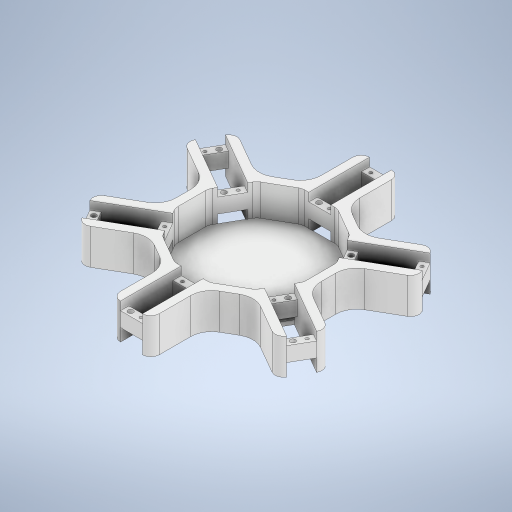
# Autodesk Inventor part: HexBodyBottom
Saved by Autodesk Inventor 2024 (Build 280153000, 153)
## iProperties
Created: 2026-02-25
Part Number: HexBodyBottom
Material: Generic
Document SubType Name: Modeling
Designer: Liam
Density: 1 g/cm^3
Appearance: Default
Author: Liam
Autodesk Inventor part; units mm, degrees
ref_plane "YZ Plane" through (0, 0, 0) normal (1, 0, 0) x (0, 1, 0)
ref_plane "XZ Plane" through (0, 0, 0) normal (0, 1, 0) x (-1, 0, 0)
ref_plane "XY Plane" through (0, 0, 0) normal (0, 0, 1) x (1, 0, 0)
sketch "Sketch1" plane through (0, 0, 0) normal (0, 1, 0) x (-1, 0, 0)
  line L0 (0, -80) -> (-69.282, -40)
  line L1 (-69.282, -40) -> (-69.282, 40)
  line L2 (-69.282, 40) -> (0, 80)
  line L3 (0, 80) -> (69.282, 40)
  line L4 (69.282, 40) -> (69.282, -40)
  line L5 (69.282, -40) -> (0, -80)
  line L6 (128, 128) -> (-128, 128)
  line L7 (-128, 128) -> (-128, -128)
  line L8 (-128, -128) -> (128, -128)
  line L9 (128, -128) -> (128, 128)
  line L10 (128, 128) -> (-128, -128) construction
  line L11 (-128, 128) -> (128, -128) construction
  line L12 (10.5, 111) -> (-10.5, 111)
  line L13 (-10.5, 111) -> (-10.5, 69)
  line L14 (-10.5, 69) -> (10.5, 69)
  line L15 (10.5, 69) -> (10.5, 111)
  line L16 (10.5, 111) -> (-10.5, 69) construction
  line L17 (-10.5, 111) -> (10.5, 69) construction
  line L18 (18.5, 119) -> (-18.5, 119)
  line L19 (-18.5, 119) -> (-18.5, 61)
  line L20 (-18.5, 61) -> (18.5, 61)
  line L21 (18.5, 61) -> (18.5, 119)
  line L22 (61.282, 35.3812) -> (0, 70.7624)
  line L23 (0, 70.7624) -> (-61.282, 35.3812)
  line L24 (-61.282, 35.3812) -> (-61.282, -35.3812)
  line L25 (-61.282, -35.3812) -> (0, -70.7624)
  line L26 (0, -70.7624) -> (61.282, -35.3812)
  line L27 (61.282, -35.3812) -> (61.282, 35.3812)
  circle A0 centre (-5, 114.75) radius 1.5
  circle A1 centre (5, 114.75) radius 2.5
  circle A2 centre (5, 65.25) radius 1.5
  circle A3 centre (-5, 65.25) radius 2.5
  line L28 (-10.5, 111) -> (-10.5, 119)
  line L29 (10.5, 111) -> (10.5, 119)
  line L30 (-10.5, 69) -> (-10.5, 61)
  line L31 (10.5, 69) -> (10.5, 61)
  line L32 (-43.5775, 46.5215) -> (-93.807, 75.5215)
  line L33 (-93.807, 75.5215) -> (-112.307, 43.4785)
  line L34 (-90.8788, 64.5933) -> (-97.807, 68.5933)
  line L35 (-54.5058, 43.5933) -> (-90.8788, 64.5933)
  line L36 (-90.8788, 64.5933) -> (-101.3788, 46.4067)
  circle A4 centre (-96.8764, 61.7051) radius 2.5
  circle A5 centre (-101.8764, 53.0449) radius 1.5
  line L37 (-101.3788, 46.4067) -> (-108.307, 50.4067)
  line L38 (-101.3788, 46.4067) -> (-65.0058, 25.4067)
  line L39 (-112.307, 43.4785) -> (-62.0775, 14.4785)
  line L40 (-62.0775, 14.4785) -> (-43.5775, 46.5215)
  line L41 (-65.0058, 25.4067) -> (-58.0775, 21.4067)
  circle A6 centre (-59.0082, 28.2949) radius 2.5
  circle A7 centre (-54.0082, 36.9551) radius 1.5
  line L42 (-65.0058, 25.4067) -> (-54.5058, 43.5933)
  line L43 (-54.5058, 43.5933) -> (-47.5775, 39.5933)
  line L44 (-62.0775, -14.4785) -> (-112.307, -43.4785)
  line L45 (-112.307, -43.4785) -> (-93.807, -75.5215)
  line L46 (-101.3788, -46.4067) -> (-108.307, -50.4067)
  line L47 (-65.0058, -25.4067) -> (-101.3788, -46.4067)
  line L48 (-101.3788, -46.4067) -> (-90.8788, -64.5933)
  circle A8 centre (-101.8764, -53.0449) radius 2.5
  circle A9 centre (-96.8764, -61.7051) radius 1.5
  line L49 (-90.8788, -64.5933) -> (-97.807, -68.5933)
  line L50 (-90.8788, -64.5933) -> (-54.5058, -43.5933)
  line L51 (-93.807, -75.5215) -> (-43.5775, -46.5215)
  line L52 (-43.5775, -46.5215) -> (-62.0775, -14.4785)
  line L53 (-54.5058, -43.5933) -> (-47.5775, -39.5933)
  circle A10 centre (-54.0082, -36.9551) radius 2.5
  circle A11 centre (-59.0082, -28.2949) radius 1.5
  line L54 (-54.5058, -43.5933) -> (-65.0058, -25.4067)
  line L55 (-65.0058, -25.4067) -> (-58.0775, -21.4067)
  line L56 (-18.5, -61) -> (-18.5, -119)
  line L57 (-18.5, -119) -> (18.5, -119)
  line L58 (-10.5, -111) -> (-10.5, -119)
  line L59 (-10.5, -69) -> (-10.5, -111)
  line L60 (-10.5, -111) -> (10.5, -111)
  circle A12 centre (-5, -114.75) radius 2.5
  circle A13 centre (5, -114.75) radius 1.5
  line L61 (10.5, -111) -> (10.5, -119)
  line L62 (10.5, -111) -> (10.5, -69)
  line L63 (18.5, -119) -> (18.5, -61)
  line L64 (18.5, -61) -> (-18.5, -61)
  line L65 (10.5, -69) -> (10.5, -61)
  circle A14 centre (5, -65.25) radius 2.5
  circle A15 centre (-5, -65.25) radius 1.5
  line L66 (10.5, -69) -> (-10.5, -69)
  line L67 (-10.5, -69) -> (-10.5, -61)
  line L68 (43.5775, -46.5215) -> (93.807, -75.5215)
  line L69 (93.807, -75.5215) -> (112.307, -43.4785)
  line L70 (90.8788, -64.5933) -> (97.807, -68.5933)
  line L71 (54.5058, -43.5933) -> (90.8788, -64.5933)
  line L72 (90.8788, -64.5933) -> (101.3788, -46.4067)
  circle A16 centre (96.8764, -61.7051) radius 2.5
  circle A17 centre (101.8764, -53.0449) radius 1.5
  line L73 (101.3788, -46.4067) -> (108.307, -50.4067)
  line L74 (101.3788, -46.4067) -> (65.0058, -25.4067)
  line L75 (112.307, -43.4785) -> (62.0775, -14.4785)
  line L76 (62.0775, -14.4785) -> (43.5775, -46.5215)
  line L77 (65.0058, -25.4067) -> (58.0775, -21.4067)
  circle A18 centre (59.0082, -28.2949) radius 2.5
  circle A19 centre (54.0082, -36.9551) radius 1.5
  line L78 (65.0058, -25.4067) -> (54.5058, -43.5933)
  line L79 (54.5058, -43.5933) -> (47.5775, -39.5933)
  line L80 (62.0775, 14.4785) -> (112.307, 43.4785)
  line L81 (112.307, 43.4785) -> (93.807, 75.5215)
  line L82 (101.3788, 46.4067) -> (108.307, 50.4067)
  line L83 (65.0058, 25.4067) -> (101.3788, 46.4067)
  line L84 (101.3788, 46.4067) -> (90.8788, 64.5933)
  circle A20 centre (101.8764, 53.0449) radius 2.5
  circle A21 centre (96.8764, 61.7051) radius 1.5
  line L85 (90.8788, 64.5933) -> (97.807, 68.5933)
  line L86 (90.8788, 64.5933) -> (54.5058, 43.5933)
  line L87 (93.807, 75.5215) -> (43.5775, 46.5215)
  line L88 (43.5775, 46.5215) -> (62.0775, 14.4785)
  line L89 (54.5058, 43.5933) -> (47.5775, 39.5933)
  circle A22 centre (54.0082, 36.9551) radius 2.5
  circle A23 centre (59.0082, 28.2949) radius 1.5
  line L90 (54.5058, 43.5933) -> (65.0058, 25.4067)
  line L91 (65.0058, 25.4067) -> (58.0775, 21.4067)
  point P0 (0, 0)
  point P1 (0, 0)
  point P2 (0, 0)
  point P3 (0, 90)
  point P4 (30.641, 53.0718)
  point P5 (0, 69)
  point P6 (16.909, 61)
  point P7 (-16.909, 61)
  point P8 (-18.5, 69.319)
  point P9 (18.5, 69.319)
  point P10 (-59.7558, 34.5)
  point P11 (-59.7558, -34.5)
  point P12 (0, -69)
  point P13 (59.7558, -34.5)
  point P14 (59.7558, 34.5)
  point P15 (-69.282, 18.638)
  point P16 (-69.282, -18.638)
  point P17 (-50.782, -50.681)
  point P18 (-18.5, -69.319)
  point P19 (18.5, -69.319)
  point P20 (50.782, -50.681)
  point P21 (69.282, -18.638)
  point P22 (69.282, 18.638)
  point P23 (50.782, 50.681)
  point P24 (44.3731, 45.1436)
  point P25 (61.282, 15.8564)
  point P26 (61.282, -15.8564)
  point P27 (44.3731, -45.1436)
  point P28 (16.909, -61)
  point P29 (-16.909, -61)
  point P30 (-44.3731, -45.1436)
  point P31 (-61.282, -15.8564)
  point P32 (-61.282, 15.8564)
  point P33 (-44.3731, 45.1436)
  point P34 (-50.782, 50.681)
  point P35 (10.5, 73.9378)
  point P36 (-10.5, 73.9378)
  point P37 (-58.782, 46.0622)
  point P38 (-69.282, 27.8756)
  point P39 (-69.282, -27.8756)
  point P40 (-58.782, -46.0622)
  point P41 (-10.5, -73.9378)
  point P42 (10.5, -73.9378)
  point P43 (58.782, -46.0622)
  point P44 (69.282, -27.8756)
  point P45 (69.282, 27.8756)
  point P46 (58.782, 46.0622)
  dimension "d0" = 0
  dimension "d1" = 80
  dimension "d2" = 256
  dimension "d3" = 256
  dimension "d4" = 0
  dimension "d5" = 0
  dimension "d7" = 90
  dimension "d9" = 0
  dimension "d10" = 42
  dimension "d11" = 21
  dimension "d12" = 8
  dimension "d13" = 8
  dimension "d14" = 119
  dimension "d15" = 3
  dimension "d16" = 5
  dimension "d17" = 3.75
  dimension "d18" = 3.75
  dimension "d19" = 5
  dimension "d20" = 5
  dimension "d21" = 3
  dimension "d22" = 5
  dimension "d23" = 3.75
  dimension "d24" = 3.75
  dimension "d25" = 5
  dimension "d26" = 5
  dimension "d37" = 360
  constraints: 184 end point, 30 point on line, 24 centre point, 6 midpoint, 6 parallel, 6 perpendicular, 2 horizontal, 1 coincident, 220 other
  measures "d0" horizontal distance of L0.start point (0, 0)
  measures "d1" distance of L3.end L4.end
  measures "d2" distance of L6.start L6.end
  measures "d3" distance of L6.end L7.end
  measures "d4" distance of point (0, 0) point (0, 0)
  measures "d5" distance of point (0, 0) point (0, 0)
  measures "d7" distance of point (0, 0) point (0, 90)
  measures "d9" horizontal distance of L2.end point (0, 90)
  measures "d10" distance of L14.end L12.start
  measures "d11" distance of L13.end L14.end
  measures "d12" distance between parallel lines of L21 L15
  measures "d13" distance from line of point (30.641, 53.072) L3
  measures "d14" distance from line of point (0, 0) L18
  measures "d15" diameter of A0
  measures "d16" diameter of A1
  measures "d17" distance from line of L12 A1.centre
  measures "d18" distance from line of L12 A0.centre
  measures "d19" horizontal distance of point (0, 90) A0.centre
  measures "d20" horizontal distance of A1.centre point (0, 90)
  measures "d21" diameter of A2
  measures "d22" diameter of A3
  measures "d23" distance from line of L14 A3.centre
  measures "d24" distance from line of L14 A2.centre
  measures "d25" horizontal distance of point (0, 69) A2.centre
  measures "d26" horizontal distance of point (0, 69) A3.centre
extrude "Extrusion1" add sketch "Sketch1" along normal blind 22 contours L59 L58 L57 L56 L0 | L0 L56 L64 L25 L67 L59 | L62 L65 L26 L64 L63 L5 | L5 L63 L57 L61 L62 | L0 L51 L52 L25 L64 L56 | L67 L25 L66 | L60 L61 L57 L58 | L63 L64 L26 L76 L68 L5 | L66 L26 A14 L65 | L51 L45 L49 L50 L0 | L0 L50 L53 L25 L52 L51 | L25 L67 L64 L65 L26 A14 L66 | L25 L64 L67 | L68 L76 L26 L79 L71 L5 | L5 L71 L70 L69 L68 | L65 L64 L26 | L49 L45 L46 L48 | L54 L25 A10 L53 | L25 L53 L52 | L79 L26 L78 | L72 L73 L69 L70 | L76 L79 L26 | L47 L46 L45 L44 L1 | L1 L44 L52 L24 L55 L47 | L25 A10 L54 L24 L55 L52 L53 | L74 L77 L27 L76 L75 L4 | L4 L75 L69 L73 L74 | L26 L79 L76 L77 L27 A18 L78 | L1 L39 L40 L24 L52 L44 | L55 L24 L54 | L55 L24 L52 | L75 L76 L27 L88 L80 L4 | L78 L27 A18 L77 | L76 L27 L77 | L39 L33 L37 L38 L1 | L1 L38 L41 L24 L40 L39 | L80 L88 L27 L91 L83 L4 | L4 L83 L82 L81 L80 | L24 L41 L40 | L88 L91 L27 | L37 L33 L34 L36 | L42 L24 A6 L41 | L24 A6 L42 L23 L43 L40 L41 | L91 L27 L90 | L84 L85 L81 L82 | L91 L88 L89 L22 A22 L90 L27 | L35 L34 L33 L32 L2 | L2 L32 L40 L23 L43 L35 | L43 L23 L40 | L86 L89 L22 L88 L87 L3 | L3 L87 L81 L85 L86 | L88 L22 L89 | L2 L19 L20 L23 L40 L32 | L43 L23 L42 | L87 L88 L22 L20 L21 L3 | L90 L22 A22 L89 | L19 L18 L28 L13 L2 | L2 L13 L30 L23 L20 L19 | L23 L30 L20 | L21 L20 L22 L31 L15 L3 | L3 L15 L29 L18 L21 | L20 L31 L22 | L30 L23 A3 L14 L22 L31 L20 | L30 L14 L23 A3 | L22 L14 L31 | L28 L18 L29 L12
extrude "Extrusion2" cut sketch "Sketch1" along normal blind 8 contours L67 L25 L66 | L60 L61 L57 L58 | L66 L26 A14 L65 | L25 L67 L64 L65 L26 A14 L66 | L49 L45 L46 L48 | L54 L25 A10 L53 | L79 L26 L78 | L72 L73 L69 L70 | L25 A10 L54 L24 L55 L52 L53 | L26 L79 L76 L77 L27 A18 L78 | L55 L24 L54 | L78 L27 A18 L77 | L37 L33 L34 L36 | L42 L24 A6 L41 | L24 A6 L42 L23 L43 L40 L41 | L91 L27 L90 | L84 L85 L81 L82 | L91 L88 L89 L22 A22 L90 L27 | L43 L23 L42 | L90 L22 A22 L89 | L30 L23 A3 L14 L22 L31 L20 | L30 L14 L23 A3 | L22 L14 L31 | L28 L18 L29 L12
extrude "Extrusion3" add sketch "Sketch1" against normal blind 4 contours L59 L58 L57 L56 L0 | L0 L56 L64 L25 L67 L59 | L62 L65 L26 L64 L63 L5 | L5 L63 L57 L61 L62 | L0 L51 L52 L25 L64 L56 | L63 L64 L26 L76 L68 L5 | L51 L45 L49 L50 L0 | L0 L50 L53 L25 L52 L51 | L25 L64 L67 | L68 L76 L26 L79 L71 L5 | L5 L71 L70 L69 L68 | L65 L64 L26 | L25 L52 L24 L40 L23 L20 L22 L88 L27 L76 L26 L64 | L25 L53 L52 | L76 L79 L26 | L47 L46 L45 L44 L1 | L1 L44 L52 L24 L55 L47 | L74 L77 L27 L76 L75 L4 | L4 L75 L69 L73 L74 | L1 L39 L40 L24 L52 L44 | L55 L24 L52 | L75 L76 L27 L88 L80 L4 | L76 L27 L77 | L39 L33 L37 L38 L1 | L1 L38 L41 L24 L40 L39 | L80 L88 L27 L91 L83 L4 | L4 L83 L82 L81 L80 | L24 L41 L40 | L88 L91 L27 | L35 L34 L33 L32 L2 | L2 L32 L40 L23 L43 L35 | L43 L23 L40 | L86 L89 L22 L88 L87 L3 | L3 L87 L81 L85 L86 | L88 L22 L89 | L2 L19 L20 L23 L40 L32 | L87 L88 L22 L20 L21 L3 | L19 L18 L28 L13 L2 | L2 L13 L30 L23 L20 L19 | L23 L30 L20 | L21 L20 L22 L31 L15 L3 | L3 L15 L29 L18 L21 | L20 L31 L22
extrude "Extrusion4" add sketch "Sketch1" along normal blind 30 contours L59 L58 L57 L56 L0 | L0 L56 L64 L25 L67 L59 | L62 L65 L26 L64 L63 L5 | L5 L63 L57 L61 L62 | L0 L51 L52 L25 L64 L56 | L63 L64 L26 L76 L68 L5 | L51 L45 L49 L50 L0 | L0 L50 L53 L25 L52 L51 | L25 L64 L67 | L68 L76 L26 L79 L71 L5 | L5 L71 L70 L69 L68 | L65 L64 L26 | L25 L53 L52 | L76 L79 L26 | L47 L46 L45 L44 L1 | L1 L44 L52 L24 L55 L47 | L74 L77 L27 L76 L75 L4 | L4 L75 L69 L73 L74 | L1 L39 L40 L24 L52 L44 | L55 L24 L52 | L75 L76 L27 L88 L80 L4 | L76 L27 L77 | L39 L33 L37 L38 L1 | L1 L38 L41 L24 L40 L39 | L80 L88 L27 L91 L83 L4 | L4 L83 L82 L81 L80 | L24 L41 L40 | L88 L91 L27 | L35 L34 L33 L32 L2 | L2 L32 L40 L23 L43 L35 | L43 L23 L40 | L86 L89 L22 L88 L87 L3 | L3 L87 L81 L85 L86 | L88 L22 L89 | L2 L19 L20 L23 L40 L32 | L87 L88 L22 L20 L21 L3 | L19 L18 L28 L13 L2 | L2 L13 L30 L23 L20 L19 | L23 L30 L20 | L21 L20 L22 L31 L15 L3 | L3 L15 L29 L18 L21 | L20 L31 L22
fillet "Fillet1" radius 8 12 edges at (-93.807, 13, 75.5215) (-112.307, 13, 43.4785) (18.5, 13, 119) (93.807, 13, 75.5215) (112.307, 13, 43.4785) (112.307, 13, -43.4785) (93.807, 13, -75.5215) (18.5, 13, -119) (-18.5, 13, -119) (-93.807, 13, -75.5215) (-112.307, 13, -43.4785) (-18.5, 13, 119)
fillet "Fillet2" radius 20 12 edges at (18.5, 13, 69.319) (50.782, 13, 50.681) (69.282, 13, 18.638) (69.282, 13, -18.638) (50.782, 13, -50.681) (18.5, 13, -69.319) (-18.5, 13, -69.319) (-50.782, 13, -50.681) (-69.282, 13, -18.638) (-69.282, 13, 18.638) (-50.782, 13, 50.681) (-18.5, 13, 69.319)
fillet "Fillet3" radius 10 12 edges at (61.282, 15, -15.8564) (61.282, 15, 15.8564) (44.3731, 15, 45.1436) (16.909, 15, 61) (-16.909, 15, 61) (-44.3731, 15, 45.1436) (-61.282, 15, 15.8564) (-61.282, 15, -15.8564) (-44.3731, 15, -45.1436) (-16.909, 15, -61) (16.909, 15, -61) (44.3731, 15, -45.1436)
equation "\"d10\" = MountLength"
equation "\"d11\" = MountWidth"
equation "\"d12\" = MountThickness"
equation "\"d13\" = MountThickness"
equation "\"d15\" = HOLE_DIAMETER"
equation "\"d16\" = INSERT_DIAMETER"
equation "\"d17\" = MountHoleY"
equation "\"d18\" = MountHoleY"
equation "\"d19\" = MountHoleX"
equation "\"d20\" = MountHoleX"
equation "\"d21\" = HOLE_DIAMETER"
equation "\"d22\" = INSERT_DIAMETER"
equation "\"d23\" = MountHoleY"
equation "\"d24\" = MountHoleY"
equation "\"d25\" = MountHoleX"
equation "\"d26\" = MountHoleX"
equation "\"d27\" = OUTER_HEIGHT + INNER_HEIGHT"
equation "\"d29\" = OUTER_HEIGHT"
equation "\"d33\" = 2 * OUTER_HEIGHT + INNER_HEIGHT"
equation "\"MountLength\" = 42"
equation "\"MountWidth\" = 21"
equation "\"MountThickness\" = 8"
equation "\"HOLE_DIAMETER\" = 3"
equation "\"INSERT_DIAMETER\" = 5"
equation "\"MountHoleY\" = 3.75"
equation "\"OUTER_HEIGHT\" = 8"
equation "\"INNER_HEIGHT\" = 14"
equation "\"MountHoleX\" = 5"
body "Solid1"
